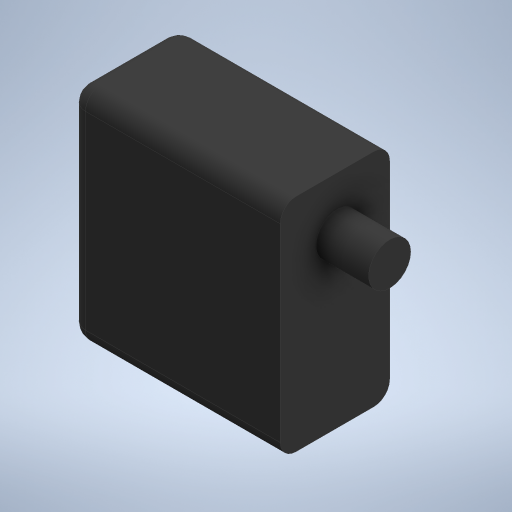
# Autodesk Inventor part: servomoteur
Saved by Autodesk Inventor 2024.1 (Build 281209000, 209)
## iProperties
Created: 2024-04-29
Part Number: servomoteur
Material: Générique
Document SubType Name: Modeling
Designer: chass
Density: 1 g/cm^3
Appearance: Par défaut
Author: chass
Autodesk Inventor part; units mm, degrees
ref_plane "YZ Plane" through (0, 0, 0) normal (1, 0, 0) x (0, 1, 0)
ref_plane "XZ Plane" through (0, 0, 0) normal (0, 1, 0) x (-1, 0, 0)
ref_plane "XY Plane" through (0, 0, 0) normal (0, 0, 1) x (1, 0, 0)
sketch "Esquisse1" plane through (0, 0, 0) normal (1, 0, 0) x (0, 1, 0)
  line L0 (10, 13.8) -> (-32, 13.8)
  line L1 (-32, 13.8) -> (-32, -7)
  line L2 (-32, -7) -> (10, -7)
  line L3 (10, -7) -> (10, 13.8)
  point P0 (0, 0)
  dimension "d0" = 42
  dimension "d1" = 20.8
  constraints: 8 end point, 2 parallel, 1 horizontal, 1 perpendicular
  measures "d0" distance of L1.end L2.end
  measures "d1" distance of L2.end L0.start
extrude "Extrusion1" add sketch "Esquisse1" along normal blind 40
sketch "Esquisse2" plane through (40, 0, 0) normal (1, 0, 0) x (0, 0, -1)
  circle A0 centre (-3, 0) radius 4
  line L0 (7, 10) -> (-13.8, 10) projected
  line L1 (-3.4, 0) -> (-13.8, 0)
  line L2 (-3, 0) -> (7, 0)
  point P0 (0, 0)
  dimension "d4" = 10
  constraints: 4 end point, 2 horizontal, 1 centre point, 1 collinear
  measures "d4" distance from line of L0 L2.start
extrude "Extrusion2" add sketch "Esquisse2" along normal blind 10
fillet "Congé1" radius 3 8 edges at (20, 10, 13.8) (20, 10, -7) (0, 10, 3.4) (0, -11, 13.8) (0, -11, -7) (0, -32, 3.4) (20, -32, 13.8) (20, -32, -7)
